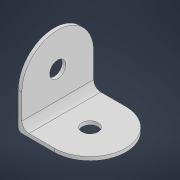
# Autodesk Inventor part: Vertical Support - 90deg Bracket
Saved by Autodesk Inventor 2022 (Build 260153000, 153)
## iProperties
Created: 2023-06-23
Part Number: Vertical Support - 90deg Bracket
Material: Generic
Document SubType Name: Modeling
Designer: Ryan Mitcham
Density: 1 g/cm^3
Appearance: Default
Author: Ryan Mitcham
Autodesk Inventor part; units mm, degrees
ref_plane "YZ Plane" through (0, 0, 0) normal (1, 0, 0) x (0, 1, 0)
ref_plane "XZ Plane" through (0, 0, 0) normal (0, 1, 0) x (-1, 0, 0)
ref_plane "XY Plane" through (0, 0, 0) normal (0, 0, 1) x (1, 0, 0)
sketch "Sketch1" plane through (0, 0, 0) normal (0, 0, 1) x (1, 0, 0)
  line L0 (0, 20) -> (0, 0)
  line L1 (0, 0) -> (20, 0)
  line L2 (20, 0) -> (20, 1)
  line L3 (20, 1) -> (1, 1)
  line L4 (1, 1) -> (1, 20)
  line L5 (1, 20) -> (0, 20)
  dimension "d0" = 20
  dimension "d1" = 20
  dimension "d2" = 1
  dimension "d3" = 1
  constraints: 12 end point, 5 perpendicular, 1 vertical
  measures "d0" distance of L0.start L0.end
  measures "d1" distance of L0.end L1.end
  measures "d2" distance of L1.end L2.end
  measures "d3" distance of L4.end L0.start
extrude "Extrusion1" add sketch "Sketch1" along normal blind 20
sketch "Sketch2" plane through (1, 1, 0) normal (1, 0, 0) x (0, 0, -1)
  line L0 (0, 19) -> (-20, 19) projected
  line L1 (0, 0) -> (0, 19) projected
  point P0 (0, -1)
  point P1 (-10, 9.5)
  point P2 (-10, 19)
  point P3 (0, 9.5)
  constraints: 2 midpoint, 1 horizontal alignment, 1 vertical alignment
hole "Hole1" at (1, 10.5, 10) direction (-1, 0, 0) diameter 4.5 end through all
sketch "Sketch3" plane through (1, 1, 0) normal (0, 1, 0) x (1, 0, 0)
  line L0 (-1, 0) -> (19, 0) projected
  line L1 (19, 0) -> (19, -20) projected
  point P0 (9, -10)
  point P1 (9, 0)
  point P2 (19, -10)
  constraints: 2 midpoint, 1 horizontal alignment, 1 vertical alignment
hole "Hole2" at (10, 1, 10) direction (0, -1, 0) diameter 4.5 end through all
fillet "Fillet1" radius 2 1 edges at (1, 1, 10)
fillet "Fillet2" radius 10 4 edges at (0.5, 20, 20) (0.5, 20, 0) (20, 0.5, 0) (20, 0.5, 20)
fillet "Fillet3" radius 1 1 edges at (0, 0, 10)
body "Solid1"
